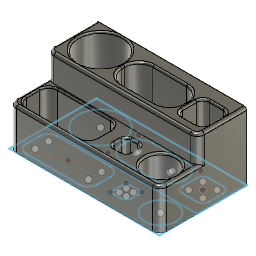
BathroomOrganizer v1 (Autodesk Fusion 360 design; units mm, degrees)
Autodesk Fusion 360 part; units mm, degrees
sketch "Sketch1" plane through (0, 0, 0) normal (0, 0, 1) x (1, 0, 0)
  line L0 (-19, 42.5) -> (19, 42.5)
  line L1 (35, 26.5) -> (35, 23.5)
  line L2 (19, 7.5) -> (-19, 7.5)
  line L3 (-35, 23.5) -> (-35, 26.5)
  arc A0 (-19, 42.5) -> (-35, 26.5) centre (-19, 26.5) ccw
  arc A1 (-35, 23.5) -> (-19, 7.5) centre (-19, 23.5) ccw
  arc A2 (19, 7.5) -> (35, 23.5) centre (19, 23.5) ccw
  arc A3 (35, 26.5) -> (19, 42.5) centre (19, 26.5) ccw
  circle A4 centre (-64.0752, 28.2939) radius 25
  line L4 (63, 10) -> (47, 10)
  line L5 (40, 17) -> (40, 33)
  line L6 (47, 40) -> (63, 40)
  line L7 (70, 33) -> (70, 17)
  line L8 (70, 10) -> (40, 40) construction
  line L9 (40, 10) -> (70, 40) construction
  arc A5 (47, 40) -> (40, 33) centre (47, 33) ccw
  arc A6 (40, 17) -> (47, 10) centre (47, 17) ccw
  arc A7 (63, 10) -> (70, 17) centre (63, 17) ccw
  arc A8 (70, 33) -> (63, 40) centre (63, 33) ccw
  line L10 (-20, -39.5) -> (-80, -39.5)
  line L11 (-90, -29.5) -> (-90, -14.5)
  line L12 (-80, -4.5) -> (-20, -4.5)
  line L13 (-10, -14.5) -> (-10, -29.5)
  line L14 (-10, -39.5) -> (-90, -4.5) construction
  line L15 (-90, -39.5) -> (-10, -4.5) construction
  arc A9 (-80, -4.5) -> (-90, -14.5) centre (-80, -14.5) ccw
  arc A10 (-90, -29.5) -> (-80, -39.5) centre (-80, -29.5) ccw
  arc A11 (-20, -39.5) -> (-10, -29.5) centre (-20, -29.5) ccw
  arc A12 (-10, -14.5) -> (-20, -4.5) centre (-20, -14.5) ccw
  line L16 (9.9672, -11.5847) -> (17.9672, -11.5847)
  line L17 (22.9672, -16.5847) -> (22.9672, -24.5847)
  line L18 (17.9672, -29.5847) -> (9.9672, -29.5847)
  line L19 (4.9672, -24.5847) -> (4.9672, -16.5847)
  arc A13 (9.9672, -11.5847) -> (4.9672, -16.5847) centre (9.9672, -16.5847) ccw
  arc A14 (22.9672, -16.5847) -> (17.9672, -11.5847) centre (17.9672, -16.5847) ccw
  arc A15 (17.9672, -29.5847) -> (22.9672, -24.5847) centre (17.9672, -24.5847) ccw
  arc A16 (4.9672, -24.5847) -> (9.9672, -29.5847) centre (9.9672, -24.5847) ccw
  circle A17 centre (53.3224, -21.2914) radius 17.5
  line L20 (-94.8686, 54.5) -> (75, 54.5)
  line L21 (75, 54.5) -> (75, -44)
  line L22 (75, -44) -> (-94.8686, -44)
  line L23 (-94.8686, -44) -> (-94.8686, 54.5)
  line L24 (-94.8686, -1.5595) -> (75, -1.5595)
  line L25 (75, -1.5595) -> (75, 54.5)
  line L26 (75, 54.5) -> (-94.8686, 54.5)
  line L27 (-94.8686, 54.5) -> (-94.8686, -1.5595)
  point P0 (-35, 42.5)
  point P1 (35, 42.5)
  point P2 (-35, 7.5)
  point P3 (55, 25)
  point P4 (-50, -22)
  point P5 (4.9672, -11.5847)
  point P6 (22.9672, -11.5847)
  point P7 (4.9672, -29.5847)
  dimension "d1" = 70
  dimension "d2" = 35
  dimension "d3" = 16
  dimension "d4" = 16
  dimension "d5" = 16
  dimension "d6" = 16
  dimension "d7" = 50
  dimension "d8" = 30
  dimension "d9" = 30
  dimension "d10" = 7
  dimension "d11" = 80
  dimension "d12" = 35
  dimension "d13" = 10
  dimension "d14" = 18
  dimension "d15" = 18
  dimension "d16" = 5
  dimension "d17" = 35
  constraint horizontal L0
  constraint vertical L1
  constraint horizontal L2
  constraint vertical L3
  constraint coincident P0 L0
  constraint coincident P0 L3
  constraint tangent L0 A0
  constraint tangent L3 A0
  constraint coincident P2 L2
  constraint coincident P2 L3
  constraint tangent L2 A1
  constraint tangent L3 A1
  constraint tangent L1 A2
  constraint tangent L2 A2
  constraint coincident P1 L1
  constraint coincident P1 L0
  constraint tangent L1 A3
  constraint tangent L0 A3
  constraint horizontal L4
  constraint perpendicular L4 L5
  constraint parallel L4 L6
  constraint parallel L5 L7
  constraint coincident L8 P3
  constraint coincident L9 P3
  constraint coincident L8.end L6
  constraint coincident L8.end L5
  constraint tangent L6 A5
  constraint tangent L5 A5
  constraint coincident L9.start L4
  constraint coincident L9.start L5
  constraint tangent L4 A6
  constraint tangent L5 A6
  constraint equal A5 A6
  constraint coincident L8.start L7
  constraint coincident L8.start L4
  constraint tangent L7 A7
  constraint tangent L4 A7
  constraint equal A5 A7
  constraint coincident L9.end L6
  constraint coincident L9.end L7
  constraint tangent L6 A8
  constraint tangent L7 A8
  constraint equal A5 A8
  constraint horizontal L10
  constraint perpendicular L10 L11
  constraint parallel L10 L12
  constraint parallel L11 L13
  constraint coincident L14 P4
  constraint coincident L15 P4
  constraint coincident L14.end L12
  constraint coincident L14.end L11
  constraint tangent L12 A9
  constraint tangent L11 A9
  constraint coincident L15.start L10
  constraint coincident L15.start L11
  constraint tangent L10 A10
  constraint tangent L11 A10
  constraint equal A9 A10
  constraint coincident L14.start L10
  constraint coincident L14.start L13
  constraint tangent L10 A11
  constraint tangent L13 A11
  constraint equal A9 A11
  constraint coincident L15.end L12
  constraint coincident L15.end L13
  constraint tangent L12 A12
  constraint tangent L13 A12
  constraint equal A9 A12
  constraint horizontal L16
  constraint vertical L17
  constraint horizontal L18
  constraint vertical L19
  constraint coincident P5 L16
  constraint coincident P5 L19
  constraint tangent L16 A13
  constraint tangent L19 A13
  constraint coincident P6 L17
  constraint coincident P6 L16
  constraint tangent L17 A14
  constraint tangent L16 A14
  constraint equal A13 A14
  constraint tangent L17 A15
  constraint tangent L18 A15
  constraint equal A13 A15
  constraint coincident P7 L19
  constraint coincident P7 L18
  constraint tangent L19 A16
  constraint tangent L18 A16
  constraint equal A13 A16
  constraint horizontal L20
  constraint vertical L21
  constraint horizontal L22
  constraint vertical L23
  constraint horizontal L24
  constraint vertical L25
  constraint horizontal L26
  constraint vertical L27
  constraint coincident L23 L24.start
  measures "d1" distance of P0 P1
  measures "d2" distance of P0 P2
  measures "d3" radius of A0
  measures "d4" radius of A1
  measures "d5" radius of A2
  measures "d6" radius of A3
  measures "d7" diameter of A4
  measures "d8" distance of L8.end L9.end
  measures "d9" distance of L9.start L8.end
  measures "d10" radius of A5
  measures "d11" distance of L14.end L15.end
  measures "d12" distance of L15.start L14.end
  measures "d13" radius of A9
  measures "d14" distance of P5 P6
  measures "d15" distance of P5 P7
  measures "d16" radius of A13
  measures "d17" diameter of A17
extrude "Extrude1" add sketch "Sketch1" along normal blind 76.2 contours L20 L21 L23 L24 L25 L26 L27
extrude "Extrude2" add sketch "Sketch1" along normal blind 46.2 contours L21 L22 L23 L24
extrude "Extrude3" add sketch "Sketch1" along normal blind 1.2 contours L0 L1 L2 L3 A0 A1 A2 A3 | A4 | L4 L5 L6 L7 A5 A6 A7 A8 | L10 L11 L12 L13 A9 A10 A11 A12 | L16 L17 L18 L19 A13 A14 A15 A16 | A17 | L20 L21 L23 L24 L25 L26 L27 | L21 L22 L23 L24
fillet "Fillet1" radius 8 4 edges at (75, -1.5595, 61.2) (-94.8686, -1.5595, 61.2) (-94.8686, -44, 23.1) (75, -44, 23.1)
fillet "Fillet2" radius 3 10 edges at (-94.8686, -14.7797, 46.2) (-92.5254, -41.6569, 46.2) (-9.9343, -44, 46.2) (72.6569, -41.6569, 46.2) (75, -14.7797, 46.2) (-94.8686, 30.4703, 76.2) (-92.5254, 0.7837, 76.2) (-9.9343, -1.5595, 76.2) (72.6569, 0.7837, 76.2) (75, 30.4703, 76.2)
fillet "Fillet3" radius 1.5 8 edges at (-12.9289, -36.5711, 46.2) (-50, -39.5, 46.2) (-87.0711, -36.5711, 46.2) (-90, -22, 46.2) (-87.0711, -7.4289, 46.2) (-50, -4.5, 46.2) (-12.9289, -7.4289, 46.2) (-10, -22, 46.2)
fillet "Fillet4" radius 2 25 edges at (30.3137, 12.1863, 76.2) (0, 7.5, 76.2) (-30.3137, 12.1863, 76.2) (-35, 25, 76.2) (-30.3137, 37.8137, 76.2) (0, 42.5, 76.2) (30.3137, 37.8137, 76.2) (35, 25, 76.2) (70, 25, 76.2) (67.9497, 12.0503, 76.2) (55, 10, 76.2) (42.0503, 12.0503, 76.2) (40, 25, 76.2) (42.0503, 37.9497, 76.2) (55, 40, 76.2) (67.9497, 37.9497, 76.2) (37.0067, -14.9632, 46.2) (22.9672, -20.5847, 46.2) (21.5027, -28.1202, 46.2) (13.9672, -29.5847, 46.2) (6.4316, -28.1202, 46.2) (4.9672, -20.5847, 46.2) (6.4316, -13.0492, 46.2) (13.9672, -11.5847, 46.2) (21.5027, -13.0492, 46.2)
fillet "Fillet5" radius 1.75 1 edges at (-87.3834, 37.3343, 76.2)
named bodies: "Bathroom Organizer"
